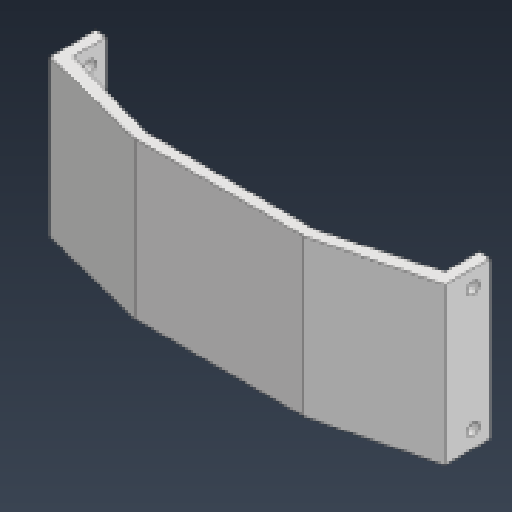
# Autodesk Inventor part: распорка шутера 1
Saved by Autodesk Inventor 2026 (Build 300175000, 175)
## iProperties
Created: 2026-01-10
Part Number: распорка шутера 1
Material: Типовые
Document SubType Name: Modeling
Designer: GameHD
Density: 1 g/cm^3
Appearance: По умолчанию
Author: GameHD
Autodesk Inventor part; units mm, degrees
ref_plane "YZ Plane" through (0, 0, 0) normal (1, 0, 0) x (0, 1, 0)
ref_plane "XZ Plane" through (0, 0, 0) normal (0, 1, 0) x (-1, 0, 0)
ref_plane "XY Plane" through (0, 0, 0) normal (0, 0, 1) x (1, 0, 0)
sketch "Эскиз1" plane through (0, 0, 0) normal (1, 0, 0) x (0, 1, 0)
  circle A0 centre (0, 0) radius 2.1
  circle A1 centre (-43, 0) radius 2.1
  line L0 (6, 20) -> (-49, 20)
  line L1 (-49, 20) -> (-49, -6)
  line L2 (-49, -6) -> (6, -6)
  line L3 (6, -6) -> (6, 20)
  point P0 (6, 7)
  dimension "d0" = 4.2
  dimension "d1" = 4.2
  dimension "d2" = 43
  dimension "d4" = 6
  dimension "d5" = 6
  dimension "d14" = 20
  dimension "d15" = 6
  constraints: 8 end point, 2 centre point, 2 parallel, 1 coincident, 1 horizontal, 1 midpoint, 1 perpendicular
  measures "d0" diameter of A0
  measures "d1" diameter of A1
  measures "d2" distance of A1.centre A0.centre
  measures "d4" distance from line of A1.centre L1
  measures "d5" distance from line of A0.centre L2
  measures "d14" distance from line of point (0, 0) L0
  measures "d15" distance from line of L3 point (0, 0)
extrude "Выдавливание1" add sketch "Эскиз1" along normal blind 4
sketch "Эскиз2" plane through (4, 0, 0) normal (1, 0, 0) x (0, 0, -1)
  line L0 (6, 6) -> (-20, 6) projected
  line L1 (-20, -49) -> (6, -49) projected
  line L2 (-20, 6) -> (-16, 6)
  line L3 (-16, 6) -> (-16, -49)
  line L4 (-16, -49) -> (-20, -49)
  line L5 (-20, -49) -> (-20, 6)
  point P0 (0, 0)
  dimension "d9" = 4
  constraints: 8 end point, 2 parallel, 1 horizontal, 1 perpendicular, 1 point on line
  measures "d9" distance between parallel lines of L5 L3
extrude "Выдавливание2" add sketch "Эскиз2" along normal blind 131
sketch "Эскиз3" plane through (135, 0, 0) normal (1, 0, 0) x (0, 0, -1)
  circle A0 centre (0, -43) radius 2.1 projected
  circle A1 centre (0, 0) radius 2.1 projected
  line L0 (-16, 6) -> (-16, -49) projected
  line L1 (-16, -49) -> (6, -49) projected
  line L2 (6, -49) -> (6, 6) projected
  line L3 (6, 6) -> (-16, 6) projected
  line L4 (-20, -49) -> (-16, -49) projected
  line L5 (-16, -49) -> (-16, 6) projected
  line L6 (-16, 6) -> (-20, 6) projected
  line L7 (-20, 6) -> (-20, -49) projected
extrude "Выдавливание3" add sketch "Эскиз3" along normal blind 4
fillet "Сопряжение1" radius 10 4 edges at (4, -21.5, 16) (135, -21.5, 16) (139, -21.5, 20) (0, -21.5, 20)
sketch "Эскиз4" plane through (0, 6, -6) normal (0, 1, 0) x (1, 0, 0)
  arc A0 (4, -12) -> (14, -22) centre (14, -12) ccw projected
  line L0 (4, -12) -> (39.5, -12)
  line L1 (39.5, -12) -> (39.5, -60.325)
  line L2 (14, -22) -> (125, -22) projected
  line L3 (4, 0) -> (4, -12) projected
  line L4 (39.5, -22) -> (4, -12)
  arc A1 (0, -16) -> (10, -26) centre (10, -16) ccw projected
  line L5 (0, -16) -> (39.5, -26)
  arc A2 (0, -16) -> (10, -26) centre (10, -16) ccw projected
  line L6 (10, -26) -> (129, -26) projected
  arc A3 (129, -26) -> (139, -16) centre (129, -16) ccw projected
  line L7 (139, 0) -> (139, -16) projected
  line L8 (135, 0) -> (139, 0) projected
  line L9 (135, 0) -> (135, -12) projected
  arc A4 (125, -22) -> (135, -12) centre (125, -12) ccw projected
  line L10 (14, -22) -> (125, -22) projected
  arc A5 (4, -12) -> (14, -22) centre (14, -12) ccw projected
  line L11 (4, 0) -> (4, -12) projected
  line L12 (0, 0) -> (4, 0) projected
  line L13 (0, 0) -> (0, -16) projected
  line L14 (10, -26) -> (129, -26) projected
  line L15 (69.5, -26) -> (69.5, -19.0711)
  arc A6 (125, -22) -> (135, -12) centre (125, -12) ccw
  line L16 (135, -12) -> (99.5, -12)
  line L17 (99.5, -12) -> (99.5, -60.325)
  line L18 (135, 0) -> (135, -12)
  line L19 (99.5, -22) -> (135, -12)
  arc A7 (129, -26) -> (139, -16) centre (129, -16) ccw
  line L20 (139, -16) -> (99.5, -26)
  arc A8 (129, -26) -> (139, -16) centre (129, -16) ccw
  arc A9 (125, -22) -> (135, -12) centre (125, -12) ccw
  line L21 (135, 0) -> (135, -12)
  line L22 (139, 0) -> (135, 0)
  line L23 (139, 0) -> (139, -16)
  point P0 (0, -6)
  point P1 (10, -26)
  point P2 (39.5, -26)
  point P3 (23.7, -22)
  point P4 (5.5937, -17.4161)
  point P5 (139, -6)
  point P6 (133.4063, -17.4161)
  point P7 (115.3, -22)
  dimension "d17" = 35.5
  constraints: 26 end point, 19 symmetric about line, 8 point on circle, 5 point on line, 4 centre point, 1 horizontal, 1 midpoint, 1 perpendicular, 1 vertical, 4 other
  measures "d17" distance of L0.start L0.end
extrude "Выдавливание4" cut sketch "Эскиз4" against normal through all contours A0 L2 L5 L6 A1 | L20 L2 A4 A3 L6
sketch "Эскиз5" plane through (135, 6, -6) normal (0, 1, 0) x (1, 0, 0)
  line L0 (-135, -16) -> (-95.5, -26) projected
  line L1 (-95.5, -22) -> (-131, -12) projected
  line L2 (-111.3, -22) -> (-95.5, -26) projected
  line L3 (-95.5, -26) -> (-35.5, -26) projected
  line L4 (4, 0) -> (4, -16) projected
  line L5 (0, 0) -> (4, 0) projected
  line L6 (0, 0) -> (0, -12) projected
  arc A0 (-1.5937, -17.4161) -> (0, -12) centre (-10, -12) ccw projected
  line L7 (-111.3, -22) -> (-19.7, -22) projected
  line L8 (-135, -16) -> (-129.4063, -17.4161) projected
  arc A1 (-131, -12) -> (-129.4063, -17.4161) centre (-121, -12) ccw projected
  line L9 (-131, 0) -> (-131, -12) projected
  line L10 (-135, 0) -> (-131, 0) projected
  line L11 (-135, 0) -> (-135, -16) projected
  line L12 (-35.5, -26) -> (-19.7, -22) projected
  line L13 (-1.5937, -17.4161) -> (4, -16) projected
  line L14 (-65.5, -26) -> (-65.5, -22)
  line L15 (4, -16) -> (-35.5, -26)
  line L16 (-35.5, -22) -> (0, -12)
  point P0 (-135, -6)
  constraints: 6 end point, 4 symmetric about line, 2 midpoint
extrude "Выдавливание5" add sketch "Эскиз5" against normal up to surface (55 mm away) contours A1 L1 L7 L0 | L16 A0 L15 L7
fillet "Сопряжение2" radius 2 8 edges at (4, -21.5, 6) (0, -21.5, 10) (135, -21.5, 6) (139, -21.5, 10) (99.5, -21.5, 16) (39.5, -21.5, 16) (39.5, -21.5, 20) (99.5, -21.5, 20)
fillet "Сопряжение3" radius 4 4 edges at (137, 6, -6) (137, -49, -6) (2, -49, -6) (2, 6, -6)
